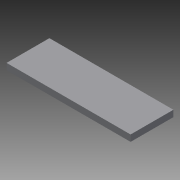
# Autodesk Inventor part: stock1
Saved by Autodesk Inventor 2015 (Build 190159000, 159)
## iProperties
Created: 2014-07-27
Part Number: stock1
Material: Generic
Document SubType Name: Modeling
Designer: pc
Density: 1 g/cm^3
Appearance: Default
Author: pc
Autodesk Inventor part; units mm, degrees
ref_plane "YZ Plane" through (0, 0, 0) normal (1, 0, 0) x (0, 1, 0)
ref_plane "XZ Plane" through (0, 0, 0) normal (0, 1, 0) x (-1, 0, 0)
ref_plane "XY Plane" through (0, 0, 0) normal (0, 0, 1) x (1, 0, 0)
sketch "Sketch1" plane through (0, 0, 0) normal (0, 0, 1) x (1, 0, 0)
  line L0 (-110, -38) -> (110, -38)
  line L1 (110, -38) -> (110, 38)
  line L2 (110, 38) -> (-110, 38)
  line L3 (-110, 38) -> (-110, -38)
  line L4 (-110, -38) -> (110, 38) construction
  line L5 (110, -38) -> (-110, 38) construction
  point P0 (0, 0)
  dimension "d0" = 220
  dimension "d1" = 76
  constraints: 12 end point, 2 midpoint, 2 parallel, 1 horizontal, 1 perpendicular
  measures "d0" distance of L1.end L2.end
  measures "d1" distance of L2.end L0.start
extrude "Extrusion1" add sketch "Sketch1" along normal blind 11.3
body "Solid1"
